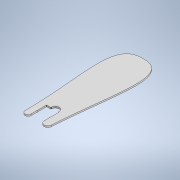
# Autodesk Inventor part: Board
Saved by Autodesk Inventor 2021 (Build 250183000, 183)
## iProperties
Created: 2021-03-08
Part Number: Board
Material: Generic
Document SubType Name: Modeling
Designer: bl17
Density: 1 g/cm^3
Appearance: Default
Author: bl17
Autodesk Inventor part; units mm, degrees
ref_plane "YZ Plane" through (0, 0, 0) normal (1, 0, 0) x (0, 1, 0)
ref_plane "XZ Plane" through (0, 0, 0) normal (0, 1, 0) x (-1, 0, 0)
ref_plane "XY Plane" through (0, 0, 0) normal (0, 0, 1) x (1, 0, 0)
sketch "Sketch2" plane through (0, 0, 0) normal (0, 1, 0) x (-1, 0, 0)
  line L0 (234.2855, -524.809) -> (-83.2145, -524.809) construction
  line L1 (-45.1145, -728.3081) -> (196.1855, -728.3081) construction
  spline S0 degree 3 poles (75.5355, -778.9546) (334.3904, -786.438) (199.8382, -405.2645) (196.6478, 110.3728) knots 0 0 0 0 1 1 1 1
  spline S1 degree 3 poles (75.5355, -778.9546) (-181.3914, -786.5378) (-57.8847, -404.3657) (-24.3239, 110.3728) knots 0 0 0 0 1 1 1 1
  line L2 (75.5355, -778.9546) -> (335.8214, -778.9546) construction
  line L3 (145.3855, 110.3728) -> (145.3855, 62.7478)
  line L4 (209.9876, 110.3728) -> (-95.098, 110.3728) construction
  arc A0 (145.3855, 62.7478) -> (145.3855, 56.3978) centre (145.3855, 59.5728) ccw
  line L5 (95.95, -54.7272) -> (55.121, -54.7272) construction
  line L6 (95.95, -54.7272) -> (136.779, -54.7272) construction
  line L7 (75.5355, -834.1569) -> (75.5355, 198.7241) construction
  line L8 (145.3855, 56.3978) -> (145.3855, -16.6272)
  line L9 (145.3855, 62.7478) -> (145.3855, 56.3978) construction
  line L10 (235, 142.3541) -> (-119.1276, 142.3541) construction
  line L11 (235, 142.3541) -> (589.1276, 142.3541) construction
  arc A1 (196.6478, 110.3728) -> (145.3855, 110.3728) centre (171.0167, 116.0926) ccw
  arc A2 (37.4355, 110.3728) -> (-24.3239, 110.3728) centre (6.5558, 111.4555) ccw
  arc A3 (37.4355, 56.3978) -> (37.4355, 62.7478) centre (37.4355, 59.5728) ccw
  line L12 (37.4355, 62.7478) -> (37.4355, 56.3978) construction
  line L13 (37.4355, 62.7478) -> (43.7855, 62.7478) construction
  line L14 (37.4355, 56.3978) -> (37.4355, -16.6272)
  line L15 (37.4355, 110.3728) -> (37.4355, 62.7478)
  line L16 (106.3264, -22.9772) -> (31.4919, -22.9772) construction
  line L17 (106.3264, -22.9772) -> (106.3264, -22.9772) construction
  arc A4 (43.7855, -22.9772) -> (107.2855, -22.9772) centre (75.5355, -22.9772) ccw
  line L18 (107.2855, -22.9772) -> (43.7855, -22.9772) construction
  line L19 (107.2855, -22.9772) -> (170.7855, -22.9772) construction
  line L20 (145.3855, -16.6272) -> (107.2855, -16.6272)
  line L21 (107.2855, -16.6272) -> (107.2855, -22.9772)
  line L22 (43.7855, -22.9772) -> (43.7855, -16.6272)
  line L23 (43.7855, -22.9772) -> (50.1355, -22.9772) construction
  line L24 (43.7855, -16.6272) -> (37.4355, -16.6272)
  point P0 (75.5355, -524.809)
  point P1 (5.0659, 158.3555)
  point P2 (75.5355, -728.3081)
  point P3 (75.5355, -35.4026)
  point P4 (75.5355, -54.7272)
  dimension "d20" = 317.5
  dimension "d37" = 241.3
  dimension "d51" = 6.35
  dimension "d52" = 50.8
  dimension "d60" = 180
  dimension "d61" = 114.3
  dimension "d76" = 180
  dimension "d81" = 6.35
  dimension "d82" = 90
  dimension "d83" = 3.175
  dimension "d84" = 50.8
  dimension "d85" = 69.85
  dimension "d86" = 38.1
  dimension "d98" = 63.5
  dimension "d99" = 180
  dimension "d100" = 31.75
  dimension "d101" = 90
  dimension "d102" = 76.2
  constraints: 51 end point, 13 horizontal, 11 point on circle, 11 point on line, 5 centre point, 5 equal length, 5 vertical, 3 midpoint, 2 collinear, 2 tangent, 1 perpendicular, 8 other
  measures "d20" distance of L0.start L0.end
  measures "d37" distance of L1.start L1.end
  measures "d51" diameter of A0
  measures "d52" distance of L3.start A0.centre
  measures "d60" angle of L5 L6
  measures "d61" distance from line of L5 A0.centre
  measures "d76" angle of L10 L11
  measures "d81" distance of L12.start L12.end
  measures "d82" angle of L12 L13
  measures "d83" radius of A3
  measures "d84" distance of L15.start A3.centre
  measures "d85" distance between parallel lines of L7 L3
  measures "d86" distance between parallel lines of L7 L15
  measures "d98" distance of L18.start L18.end
  measures "d99" angle of L18 L19
  measures "d100" radius of A4
  measures "d101" angle of L23 L22
  measures "d102" distance from line of L20 A0.centre
extrude "Extrusion1" add sketch "Sketch2" along normal blind 12.7
fillet "Fillet1" radius 3.175 4 edges at (-107.2855, 6.35, -16.6272) (-43.7855, 6.35, -16.6272) (-145.3855, 6.35, -16.6272) (-37.4355, 6.35, -16.6272)
equation "\"d37\" = d19 + 2 * d35"
equation "\"d19\" = 139.7"
equation "\"d35\" = 50.8"
body "Solid1"
